beacon_v4 (Autodesk Fusion 360 design; units mm, degrees)
Autodesk Fusion 360 part; units mm, degrees
note: some values were not read from the file. Set by a fixed rule: which sketch regions a step uses.
sketch "Esquisse1" plane through (0, 0, 0) normal (0, 0, 1) x (1, 0, 0) in component "Support"
  circle A0 centre (0, 0) radius 37.4
  circle A1 centre (0, 0) radius 42.6
  line L0 (0, 0) -> (0, 42.6) construction
  line L1 (0, -42.8) -> (0, 42.6) construction
  dimension "d1" = 74.8
  dimension "d2" = 5.2
  dimension "d4" = 85.4
  constraint coincident A0.centre A1.centre
  constraint coincident A1 L0.end
  constraint vertical L0
  constraint vertical L1
  measures "d1" diameter of A0
  measures "d4" distance of L0.end L1.start
extrude "Extrusion1" add sketch "Esquisse1" along normal blind 5 makes body 1 in component "Support"
extrude "Extrusion2" add sketch "Esquisse1" along normal blind 30 bodies 1 in component "Support"
sketch "Esquisse1 (2)" plane through (0, 0, 0) normal (0, 0, 1) x (1, 0, 0) in component "Balise"
  circle A0 centre (0, 0) radius 37.1
  circle A1 centre (0, 0) radius 32.1
  dimension "d25" = 74.2
  dimension "d26" = -5
  constraint coincident A0.centre A1.centre
  measures "d25" diameter of A0
extrude "Extrusion1'" add sketch "Esquisse1 (2)" along normal blind 80 separate body makes body 2 in component "Balise"
sketch "Esquisse3" plane through (0, 0, 80) normal (0, 0, 1) x (-1, 0, 0) in component "Balise"
  circle A0 centre (0, 0) radius 32.1
  circle A1 centre (0, 0) radius 37.1
  circle A2 centre (0, 0) radius 32.1
  dimension "d57" = 64.2
  constraint coincident A0.centre A1.centre
  measures "d57" diameter of A2
extrude "Extrusion4" add sketch "Esquisse3" against normal blind 3 contours A0 A2 bodies 2 in component "Balise"
ref_plane "Plan de construction1" through (0, -42.6, 14.8251) normal (0, -1, 0) x (-1, 0, 0) in component "Support"
sketch "Esquisse1 (3)" plane through (0, -42.6, 14.0943) normal (0, -1, 0) x (1, 0, 0) in component "Support"
  circle A0 centre (0, 5.9057) radius 2.5
  line L0 (42.6, -14.0943) -> (-42.6, -14.0943)
  line L1 (0, -14.0943) -> (0, 5.9057) construction
  point P0 (0, -14.0943)
  dimension "d42" = 5
  dimension "d43" = 20
  constraint coincident P0 L1.start
  constraint coincident A0.centre L1.end
  constraint vertical L1
  measures "d42" diameter of A0
  measures "d43" distance of A0.centre L0
ref_plane "Plan de construction2" through (0, 42.6, 15.883) normal (0, 1, 0) x (1, 0, 0) in component "Support"
sketch "Esquisse2" plane through (0, 42.6, 15.8457) normal (0, 1, 0) x (1, 0, 0) in component "Support"
  circle A0 centre (0, -4.1543) radius 2.5
  line L0 (-42.6, 15.8457) -> (42.6, 15.8457)
  line L1 (0, -4.1543) -> (0, 15.8457) construction
  dimension "d39" = 5
  dimension "d40" = 20
  constraint coincident A0.centre L1.start
  constraint midpoint L0 L1.end
  constraint perpendicular L0 L1
  measures "d39" diameter of A0
  measures "d40" distance of A0.centre L0
extrude "Extrusion1''" cut sketch "Esquisse1 (3)" against normal blind 5 bodies 1 in component "Support"
extrude "Extrusion2'" cut sketch "Esquisse2" against normal blind 5 bodies 1 in component "Support"
component "Support" placed x (1, 0, 0) y (0, 1, 0) z (0, 0, 1) at (0, 0, 0)
component "Balise" placed x (1, 0, 0) y (0, 1, 0) z (0, 0, 1) at (0, 0, 0)
equation "d4 = 75 mm + 2 * d2"
equation "d57 = 74.2 mm - 10 mm"
